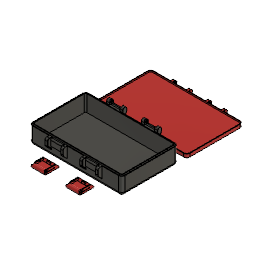
Milwaukee Tool Box Double Lock (Autodesk Fusion 360 design; units mm, degrees)
part number: 2025-08-27-12-33-30-467
Autodesk Fusion 360 part; units mm, degrees
note: some values were not read from the file. Chosen so that the rebuilt part matches the saved one: which bodies a step acts on; that a step has no effect; which face or edge a step refers to. Set by a fixed rule: which sketch regions a step uses.
sketch "Box" plane through (0, 0, 0) normal (0, 0, 1) x (1, 0, 0)
  line L0 (65.5, 43) -> (-65.5, 43)
  line L1 (-70.5, 38) -> (-70.5, -38)
  line L2 (-65.5, -43) -> (65.5, -43)
  line L3 (70.5, -38) -> (70.5, 38)
  line L4 (70.5, 43) -> (-70.5, -43) construction
  line L5 (-70.5, 43) -> (70.5, -43) construction
  arc A0 (-65.5, 43) -> (-70.5, 38) centre (-65.5, 38) ccw
  arc A1 (70.5, 38) -> (65.5, 43) centre (65.5, 38) ccw
  arc A2 (65.5, -43) -> (70.5, -38) centre (65.5, -38) ccw
  arc A3 (-70.5, -38) -> (-65.5, -43) centre (-65.5, -38) ccw
  line L6 (65.5, 40) -> (-65.5, 40)
  arc A4 (-65.5, 40) -> (-67.5, 38) centre (-65.5, 38) ccw
  line L7 (-67.5, 38) -> (-67.5, -38)
  arc A5 (-67.5, -38) -> (-65.5, -40) centre (-65.5, -38) ccw
  line L8 (-65.5, -40) -> (65.5, -40)
  arc A6 (65.5, -40) -> (67.5, -38) centre (65.5, -38) ccw
  line L9 (67.5, -38) -> (67.5, 38)
  arc A7 (67.5, 38) -> (65.5, 40) centre (65.5, 38) ccw
  line L10 (-68.5, 38) -> (-68.5, -38)
  arc A8 (-68.5, -38) -> (-65.5, -41) centre (-65.5, -38) ccw
  line L11 (-65.5, -41) -> (65.5, -41)
  arc A9 (65.5, -41) -> (68.5, -38) centre (65.5, -38) ccw
  line L12 (68.5, -38) -> (68.5, 38)
  arc A10 (68.5, 38) -> (65.5, 41) centre (65.5, 38) ccw
  line L13 (65.5, 41) -> (-65.5, 41)
  arc A11 (-65.5, 41) -> (-68.5, 38) centre (-65.5, 38) ccw
  dimension "d5" = 141
  dimension "d6" = 86
  dimension "d7" = 5
  dimension "d10" = -3
  dimension "d95" = 1
  constraint horizontal L0
  constraint perpendicular L0 L1
  constraint parallel L0 L2
  constraint parallel L1 L3
  constraint coincident L4 origin
  constraint coincident L5 origin
  constraint coincident L5.start L0
  constraint coincident L5.start L1
  constraint tangent L0 A0
  constraint tangent L1 A0
  constraint coincident L4.start L0
  constraint coincident L4.start L3
  constraint tangent L0 A1
  constraint tangent L3 A1
  constraint coincident L5.end L3
  constraint coincident L5.end L2
  constraint tangent L3 A2
  constraint tangent L2 A2
  constraint equal A1 A2
  constraint coincident L4.end L2
  constraint coincident L4.end L1
  constraint tangent L2 A3
  constraint tangent L1 A3
  constraint equal A0 A1
  constraint equal A0 A3
  measures "d5" distance of L4.end L5.end
  measures "d6" distance of L5.start L4.end
  measures "d7" radius of A0
extrude "Extrude1" add sketch "Box" along normal blind 26 contours L0 L1 L2 L3 A0 A1 A2 A3 makes body 1
extrude "Extrude15" add sketch "Box" along normal blind 27 contours L10 A8 L11 A9 L12 A10 L13 A11 bodies 1
extrude "Extrude2" add sketch "Box" along normal blind 2 contours L6 A4 L7 A5 L8 A6 L9 A7 bodies 1
chamfer "Chamfer7" distance 0.99 angle 45 8 edges at (0, -41, 26) (-67.6213, -40.1213, 26) (-68.5, 0, 26) (-67.6213, 40.1213, 26) (0, 41, 26) (67.6213, 40.1213, 26) (68.5, 0, 26) (67.6213, -40.1213, 26) on bodies 1
chamfer "Chamfer1" distance 3 angle 45 8 edges at (0, -43, 0) (69.0355, -41.5355, 0) (70.5, 0, 0) (69.0355, 41.5355, 0) (0, 43, 0) (-69.0355, 41.5355, 0) (-70.5, 0, 0) (-69.0355, -41.5355, 0) on bodies 1
fillet "Fillet1" radius 4 8 edges at (-69.0355, 41.5355, 3) (0, 43, 3) (69.0355, 41.5355, 3) (70.5, 0, 3) (69.0355, -41.5355, 3) (0, -43, 3) (-69.0355, -41.5355, 3) (-70.5, 0, 3) on bodies 1
sketch "Lid" plane through (0, 0, 26) normal (0, 0, 1) x (-1, 0, 0)
  arc A0 (70.5, 38) -> (65.5, 43) centre (65.5, 38) ccw
  line L0 (65.5, 43) -> (-65.5, 43)
  arc A1 (-65.5, 43) -> (-70.5, 38) centre (-65.5, 38) ccw
  line L1 (-70.5, 38) -> (-70.5, -38)
  arc A2 (-70.5, -38) -> (-65.5, -43) centre (-65.5, -38) ccw
  line L2 (-65.5, -43) -> (65.5, -43)
  arc A3 (65.5, -43) -> (70.5, -38) centre (65.5, -38) ccw
  line L3 (70.5, -38) -> (70.5, 38)
  arc A4 (65.5, -43) -> (70.5, -38) centre (65.5, -38) ccw
  line L4 (-65.5, -43) -> (65.5, -43)
  line L5 (70.5, -38) -> (70.5, 38)
  arc A5 (70.5, 38) -> (65.5, 43) centre (65.5, 38) ccw
  line L6 (65.5, 43) -> (-65.5, 43)
  arc A6 (-65.5, 43) -> (-70.5, 38) centre (-65.5, 38) ccw
  line L7 (-70.5, 38) -> (-70.5, -38)
  arc A7 (-70.5, -38) -> (-65.5, -43) centre (-65.5, -38) ccw
  line L8 (69.6, -38) -> (69.6, 38)
  arc A8 (69.6, 38) -> (65.5, 42.1) centre (65.5, 38) ccw
  line L9 (65.5, 42.1) -> (-65.5, 42.1)
  arc A9 (-65.5, 42.1) -> (-69.6, 38) centre (-65.5, 38) ccw
  line L10 (-69.6, 38) -> (-69.6, -38)
  arc A10 (-69.6, -38) -> (-65.5, -42.1) centre (-65.5, -38) ccw
  line L11 (-65.5, -42.1) -> (65.5, -42.1)
  arc A11 (65.5, -42.1) -> (69.6, -38) centre (65.5, -38) ccw
  arc A12 (-69.49, -38) -> (-65.5, -41.99) centre (-65.5, -38) ccw
  dimension "d18" = -0.9
extrude "Extrude3" add sketch "Lid" along normal blind 6 separate body contours A0 L0 A1 L1 A2 L2 A3 L3 A4 L4 L5 A5 L6 A6 L7 A7 | L8 A8 L9 A9 L10 A10 L11 A11 makes body 2
extrude "Extrude16" cut sketch "Lid" along normal blind 1 contours L8 A8 L9 A9 L10 A10 L11 A11 bodies 2
chamfer "Chamfer8" distance 1 angle 45 16 edges at (-68.3991, 40.8991, 27) (-69.6, 0, 27) (-68.3991, -40.8991, 27) (0, -42.1, 27) (68.3991, -40.8991, 27) (69.6, 0, 27) (68.3991, 40.8991, 27) (0, 42.1, 27) (0, -43, 32) (69.0355, -41.5355, 32) (70.5, 0, 32) (69.0355, 41.5355, 32) (0, 43, 32) (-69.0355, 41.5355, 32) (-70.5, 0, 32) (-69.0355, -41.5355, 32) on bodies 2
sketch "Lid Hinge and Latch" plane through (0, 0, 0) normal (1, 0, 0) x (0, 1, 0)
  circle A0 centre (46.2, 29) radius 1.8
  line L0 (43, 26) -> (46.2, 26)
  circle A1 centre (-46.2, 29) radius 1.8 construction
  line L1 (-44.8771, 27.5) -> (-43.9639, 27)
  circle A2 centre (-46.2, 29) radius 2
  circle A3 centre (-46.2, 29) radius 3
  line L2 (-44.8771, 30.5) -> (-43.9639, 31)
  line L3 (-49.2, 29) -> (-49.2, 9)
  line L4 (-49.2, 9) -> (-47.7, 9)
  line L5 (-47.7, 9) -> (-43, 13.7)
  line L6 (-43, 13.7) -> (-43, 26.4722)
  line L7 (-46.5, 26.015) -> (-46.5, 15.7)
  line L8 (-46.5, 15.7) -> (-43.5, 15.7)
  line L9 (-46, 15.7) -> (-46, 26.0067)
  line L10 (-43.9639, 27) -> (-43, 26.4722)
  line L11 (-43.5, 15.7) -> (-43, 15.2)
  line L12 (-46.5, 15.7) -> (-43.75, 12.95)
  line L13 (43, 26) -> (43, 31)
  line L14 (-43, 4.6569) -> (-43, 26)
  line L15 (43, 4.6569) -> (43, 26)
  line L16 (-49.2, 29) -> (-49.2, 30.2426)
  line L17 (-49.2, 30.2426) -> (-48.3213, 31.1213)
  line L18 (-38, 0) -> (-40, 0)
  line L19 (42, 32) -> (47, 32)
  line L20 (47, 32) -> (47.6938, 31.6017)
  line L21 (43, 31) -> (42, 32)
  circle A4 centre (46.2, 29) radius 3
  line L22 (-43, 26) -> (-43, 31)
  point P0 (-43, 26.4722)
  point P1 (-38, 0)
  point P2 (42, 32)
  dimension "d37" = 3.6
  dimension "d110" = 3.6
  dimension "d111" = 6
  dimension "d112" = 4
  dimension "d113" = 4
  dimension "d114" = 3
  dimension "d120" = 45
  dimension "d121" = 1.5
  dimension "d124" = 3
  dimension "d130" = 0.5
  dimension "d131" = 2
  dimension "d132" = 45
  dimension "d133" = 0.5
  dimension "d277" = 1.2426
  dimension "d337" = 89.2
  dimension "d342" = 29
  dimension "d343" = 9
  dimension "d353" = 5
  dimension "d354" = 29.863
  dimension "d355" = 6
  dimension "d356" = 89.2
  constraint coincident L1.end A3
  constraint coincident L2.end A3
  constraint concentric A1 A2
  constraint coincident L1.start A2
  constraint coincident A1.centre A2.centre
  constraint coincident L2.start A2
  constraint vertical L1.start L2.start
  constraint vertical L2.end L1.end
  constraint vertical L3
  constraint tangent A3 L3
  constraint perpendicular L3 L4
  constraint perpendicular L4 L6
  constraint vertical L7
  constraint vertical L9
  constraint parallel L1 L10
  constraint coincident A3 L7.start
  constraint coincident A3 L9.end
  constraint horizontal L8
  constraint coincident L9.start L8
  constraint coincident L6 L11.end
  constraint coincident L5 L12.end
  constraint perpendicular L5 L12
  constraint coincident A3 L3.start
  constraint coincident P0 L6.end
  constraint coincident P0 L14
  constraint coincident L0.start L13.start
  constraint perpendicular L0 L13
  constraint parallel L3 L16
  constraint coincident A3 L17.end
  constraint coincident L3.start L16.start
  constraint tangent A3 L17
  constraint horizontal L19
  constraint coincident P2 L19.start
  constraint concentric A0 A4
  constraint coincident L0.end A4
  constraint tangent L0 A4
  constraint coincident L20.end A4
  constraint tangent L20 A4
  measures "d37" diameter of A0
  measures "d110" diameter of A1
  measures "d111" diameter of A3
  measures "d112" distance of L2.end L1.end
  measures "d113" diameter of A2
  measures "d114" distance of L1.start L2.start
  measures "d120" angle of L4 L5
  measures "d121" distance of L3.end L4.end
  measures "d124" distance of L6 L9
  measures "d130" distance of L7.end L9.start
  measures "d131" distance of L5.end L8
  measures "d132" angle of L6 L11
  measures "d133" distance of L6 L8.end
  measures "d277" distance of L3.start L16.end
  measures "d337" distance of A1.centre L15
  measures "d342" distance of A1.centre L18
  measures "d343" distance of L4 L18
  measures "d353" distance of P2 L19.end
  measures "d354" angle of L19 L20
  measures "d355" diameter of A4
  measures "d356" distance of A0.centre L22
extrude "Extrude7" add sketch "Lid Hinge and Latch" along normal mid plane 15 from surface at 26.5 separate body contours L0 L13 L19 L21 A4 | A4 | L19 L20 A4 makes body 3
extrude "Extrude8" add sketch "Lid Hinge and Latch" along normal mid plane 18 from surface at 26.5 contours A0 bodies 3
chamfer "Chamfer2" distance 0.5 angle 45 2 faces at (17.5, 46.1024, 28.7514) (35.5, 46.1024, 28.7514) on bodies 3
sketch "Lid Hinge Cut" plane through (0, 43, 0) normal (0, 1, 0) x (-1, 0, 0)
  line L0 (-65.5, 26) -> (65.5, 26)
  line L1 (65.5, 26) -> (65.5, 31)
  line L2 (-65.5, 31) -> (-65.5, 26)
  line L3 (-34, 30.8) -> (-35.5, 29.934) construction
  line L4 (-35.5, 29.934) -> (-35.5, 30.8) construction
  line L5 (-35.5, 30.8) -> (-34, 30.8) construction
  line L6 (-19, 30.8) -> (-17.5, 29.934) construction
  line L7 (-17.5, 29.934) -> (-17.5, 30.8) construction
  line L8 (-17.5, 30.8) -> (-19, 30.8) construction
  line L9 (-35, 30.8) -> (-35, 27.2)
  line L10 (-18, 27.2) -> (-18, 30.8)
  line L11 (-35.5, 27.7) -> (-35.5, 30.3)
  line L12 (-17.5, 30.3) -> (-17.5, 27.7)
  line L13 (65.5, 31) -> (-65.5, 31)
  line L14 (-19, 26) -> (-19, 31)
  line L15 (-34, 31) -> (-34, 26)
  line L16 (-29, 32) -> (-24, 32)
  line L17 (-24, 32) -> (-24, 26)
  line L18 (-24, 26) -> (-29, 26)
  line L19 (-29, 26) -> (-29, 32)
  line L20 (-19, 32) -> (-34, 32)
  dimension "d357" = 30
  dimension "d358" = 30
  dimension "d365" = 5
  dimension "d366" = 5
  constraint perpendicular L0 L4
  constraint perpendicular L4 L5
  constraint perpendicular L0 L7
  constraint perpendicular L7 L8
  constraint coincident L3.end L11
  constraint coincident L6.end L12
  constraint coincident L3.start L15
  constraint coincident L6.start L14
  constraint coincident L5 L9.start
  constraint coincident L8 L10.end
  constraint horizontal L16
  constraint vertical L17
  constraint horizontal L18
  constraint vertical L19
  constraint coincident L0 L17.end
  constraint coincident L16.start L20
  measures "d357" angle of L3 L5
  measures "d358" angle of L6 L8
  measures "d365" distance of L17 L20.start
  measures "d366" distance of L16.start L20.end
extrude "Extrude40" cut sketch "Lid Hinge Cut" along normal through all contours L0 L13 L17 L18 L19 | L13 L16 L17 L19 L20 bodies 3
extrude "Extrude26" add sketch "Lid Hinge and Latch" along normal mid plane 20 from surface at 26.5 separate body contours L1 A2 A3 L2 | A3 L6 L8 L9 L10 L11 L14 L22 | A3 L3 L4 L5 L7 L12 | L5 L6 L8 L11 L12 L14 | A3 L16 L17 picked at (-44.3747, 30.9359) makes body 4
extrude "Extrude27" add sketch "Lid Hinge and Latch" along normal mid plane 17 from surface at 26.5 contours A2 bodies 4
extrude "Extrude28" add sketch "Lid Hinge and Latch" along normal mid plane 18 from surface at 26.5 contours L1 A2 A3 L2 | L1 A2 A3 L2 bodies 4
chamfer "Chamfer14" distance 0.49 angle 45 2 edges at (35, -48.0647, 29.7232) (18, -48.0647, 29.7232) on bodies 4
chamfer "Chamfer15" distance 0.5 angle 45 2 edges at (35.5, -43.2, 29) (17.5, -43.2, 29) on bodies 4
extrude "Extrude29" cut sketch "Lid Hinge and Latch" along normal mid plane 17 from surface at 26.5 contours A3 L6 L8 L9 L10 L11 L14 L22 | L5 L6 L8 L11 L12 L14 bodies 4
extrude "Extrude30" add sketch "Lid Hinge and Latch" along normal mid plane 5 from surface at 26.5 contours L5 L6 L8 L11 L12 L14 bodies 4
chamfer "Chamfer18" distance 0.4 angle 45 3 edges at (35, -43, 20.0861) (18, -43, 20.0861) (26.5, -49.2, 9) on bodies 4
fillet "Fillet4" radius 1 1 edges at (26.5, -47.7, 9) on bodies 4
sketch "Box and Lacth Hinge" plane through (0, 0, 0) normal (1, 0, 0) x (0, 1, 0)
  line L0 (43, 26) -> (43, 18)
  line L1 (-46.2, 32) -> (-42, 32)
  line L2 (-46, 24) -> (-46, 16.2)
  line L3 (-45.5, 15.7) -> (-43, 15.7)
  line L4 (-43, 9) -> (-43, 26)
  line L5 (-46, 16.2) -> (-45.5, 15.7)
  arc A0 (-46.2, 26) -> (-49.2, 23) centre (-46.2, 23) ccw
  line L6 (-49.2, 23) -> (-49.2, 16.8569)
  line L7 (-48.0284, 14.0284) -> (-43, 9)
  line L8 (-45.5, 15.7) -> (-43, 13.2)
  line L9 (43.2, 26) -> (43.2, 29)
  line L10 (48.0284, 23.0284) -> (43, 18)
  arc A1 (-49.2, 16.8569) -> (-48.0284, 14.0284) centre (-45.2, 16.8569) ccw
  circle A2 centre (-46.2, 29) radius 3
  line L11 (-43, 26) -> (-46.2, 26)
  arc A3 (-44, 26) -> (-46, 24) centre (-44, 24) ccw
  line L12 (43, 26) -> (45.0864, 26)
  line L13 (-43, 26) -> (-43, 31)
  circle A4 centre (-46.2, 29) radius 1.8
  arc A5 (48.0284, 23.0284) -> (49.2, 25.8569) centre (45.2, 25.8569) ccw
  line L14 (49.2, 29) -> (49.2, 25.8569)
  circle A6 centre (46.2, 29) radius 2
  circle A7 centre (46.2, 29) radius 1.8 construction
  circle A8 centre (46.2, 29) radius 3
  line L15 (47.7, 30.3229) -> (48.2, 31.2361)
  line L16 (44.7, 30.3229) -> (44.2, 31.2361)
  circle A9 centre (46.2, 29) radius 3.2 construction
  line L17 (43, 26) -> (46.2, 26)
  line L18 (-38, 0) -> (38, 0)
  line L19 (-43, 31) -> (-42, 32)
  line L20 (-46.2, 32) -> (-47, 32)
  line L21 (-47, 32) -> (-47.6938, 31.6017)
  circle A10 centre (46.2, 29) radius 1.3
  line L22 (47.3136, 26) -> (49.2, 26)
  arc A11 (45.0864, 26) -> (47.3136, 26) centre (46.2, 29) ccw
  point P0 (-46, 15.7)
  point P1 (-46, 15.7)
  point P2 (-49.2, 29)
  point P3 (-48.8, 9)
  point P4 (43, 26)
  point P5 (43, 26)
  point P6 (43, 31)
  dimension "d136" = 0.5
  dimension "d137" = 0.5
  dimension "d140" = 3
  dimension "d150" = 45
  dimension "d182" = 45
  dimension "d239" = 4
  dimension "d244" = 3
  dimension "d252" = 2
  dimension "d270" = 4
  dimension "d309" = 3.6
  dimension "d310" = 6
  dimension "d311" = 4
  dimension "d312" = 4
  dimension "d313" = 3
  dimension "d321" = 6.4
  dimension "d352" = 18
  dimension "d363" = 0.8
  constraint vertical L2
  constraint horizontal L3
  constraint vertical L4
  constraint coincident P1 L2
  constraint coincident P1 L3
  constraint horizontal A0.end A0.centre
  constraint vertical L6
  constraint parallel L5 L8
  constraint coincident L4 L3.end
  constraint vertical L9
  constraint coincident L0.end L10.end
  constraint vertical L0
  constraint tangent L6 A1
  constraint tangent L7 A1
  constraint coincident A2 A0.start
  constraint tangent A2 L11
  constraint horizontal L11
  constraint coincident L11 A3.start
  constraint tangent L2 A3
  constraint tangent L11 A3
  constraint coincident P1 P0
  constraint coincident L4 L8.end
  constraint vertical A0.end P2
  constraint coincident L1.start A2
  constraint horizontal L1
  constraint horizontal L4.start P3
  constraint horizontal L12
  constraint coincident P5 P4
  constraint coincident L12 A11.start
  constraint tangent L10 A5
  constraint vertical L14
  constraint coincident A5.end L14.end
  constraint tangent A5 L14
  constraint coincident L15.end A8
  constraint coincident L16.end A8
  constraint concentric A6 A7
  constraint coincident L15.start A6
  constraint coincident L16.start A6
  constraint coincident L9.end A8
  constraint horizontal L9.end A6.centre
  constraint coincident L14.start A8
  constraint concentric A8 A9
  constraint horizontal L14.start A6.centre
  constraint horizontal L15.start L16.start
  constraint horizontal L16.end L15.end
  constraint vertical L1.start A2.centre
  constraint coincident A6.centre A7.centre
  constraint coincident L12 L9.start
  constraint tangent A2 L20
  constraint coincident A2 L21.end
  constraint tangent A2 L21
  constraint coincident L1.end L19.end
  constraint coincident L12.end A9
  constraint coincident A9 L22.start
  constraint coincident L14 L22.end
  constraint perpendicular L14 L22
  constraint horizontal L12.end L22.start
  constraint concentric A9 A11
  measures "d136" distance of P1 L2.end
  measures "d137" distance of P1 L3.start
  measures "d140" distance of L2 L4
  measures "d150" angle of L4 L7
  measures "d182" angle of L0 L10
  measures "d239" radius of A1
  measures "d244" radius of A0
  measures "d252" radius of A3
  measures "d270" radius of A5
  measures "d309" diameter of A7
  measures "d310" diameter of A8
  measures "d311" distance of L16.end L15.end
  measures "d312" diameter of A6
  measures "d313" distance of L15.start L16.start
  measures "d321" diameter of A9
  measures "d352" distance of L0.end L18
  measures "d363" distance of L1.start L20.end
extrude "Extrude11" add sketch "Box and Lacth Hinge" along normal mid plane 25 from surface at 26.5 separate body contours L0 L10 L12 A5 L14 L17 L22 A11 | L9 L12 A8 L17 | A6 A8 L15 L16 | L14 A8 L17 L22 A11 | A6 A8 L15 L16 | A6 | A10 makes body 5
extrude "Extrude10" cut sketch "Box and Lacth Hinge" along normal mid plane 15.4 from surface at 26.5 contours L9 L12 A8 L17 | A6 A8 L15 L16 | L14 A8 L17 L22 A11 | A6 A8 L15 L16 | L1 A2 L11 L13 L19 bodies 5
extrude "Extrude12" cut sketch "Box and Lacth Hinge" along normal mid plane 18.4 from surface at 26.5 contours A6 | A10 bodies 5
extrude "Extrude39" cut sketch "Box and Lacth Hinge" along normal mid plane 17.4 from surface at 26.5 contours A6 A8 L15 L16 picked at (44.5493, 31.0867) bodies 5
chamfer "Chamfer4" distance 0.499 angle 45 2 faces at (17.3, 47.1704, 28.4739) (35.7, 45.9397, 29.8141) on bodies 5
chamfer "Chamfer21" distance 0.5 distance2 0.5 2 edges at (17.8, 46.2, 32) (35.2, 46.2, 32) measured on face at (15.6, 43.8719, 30.892) measured on face at (37.4, 48.5281, 30.892) on bodies 5
chamfer "Chamfer3" distance 0.2 angle 45 10 edges at (14, 46.2, 32) (14, 49.2, 27.4284) (14, 48.8955, 24.3261) (14, 45.5142, 20.5142) (14, 43.2, 27.5) (39, 49.2, 27.4284) (39, 46.2, 32) (39, 43.2, 27.5) (39, 45.5142, 20.5142) (39, 48.8955, 24.3261) on bodies 5
extrude "Extrude31" add sketch "Box and Lacth Hinge" along normal mid plane 28 from surface at 26.5 separate body contours L1 A2 L11 L13 L19 | A2 | A2 L20 L21 | A4 makes body 6
extrude "Extrude32" cut sketch "Box and Lacth Hinge" along normal mid plane 20.4 from surface at 26.5 contours L1 A2 L11 L13 L19 | A2 | A2 L20 L21 bodies 6
extrude "Extrude33" cut sketch "Box and Lacth Hinge" along normal mid plane 17.4 from surface at 26.5 contours A4 bodies 6 makes body 7 at (40.5, -45.1333, 29.6667)
chamfer "Chamfer17" distance 0.5 angle 45 2 edges at (35.2, -47.8782, 28.3491) (17.8, -47.8782, 29.6509) on bodies 6 7
chamfer "Chamfer16" distance 0.2 angle 45 6 edges at (40.5, -49.0987, 28.227) (40.5, -47.3469, 31.8008) (40.5, -44.6, 26) (12.5, -49.0987, 28.227) (12.5, -44.6, 26) (12.5, -47.3469, 31.8008) on bodies 6 7
extrude "Extrude21" add sketch "Box and Lacth Hinge" along normal mid plane 28 from surface at 26.5 separate body contours L2 L4 L5 A0 L6 L7 L8 A1 L11 A3 | L2 L3 L4 L5 L11 A3 | L3 L4 L8 makes body 8
extrude "Extrude22" cut sketch "Box and Lacth Hinge" along normal mid plane 20.4 from surface at 26.5 contours L2 L4 L5 A0 L6 L7 L8 A1 L11 A3 | L2 L3 L4 L5 L11 A3 | L3 L4 L8 bodies 8 makes body 9 at (40.5, -44.6761, 16.3428)
chamfer "Chamfer11" distance 0.2 angle 45 10 edges at (12.5, -49.2, 19.9284) (12.5, -48.3213, 25.1213) (12.5, -44.6, 26) (12.5, -45.5142, 11.5142) (12.5, -48.8955, 15.3261) (40.5, -49.2, 19.9284) (40.5, -48.8955, 15.3261) (40.5, -45.5142, 11.5142) (40.5, -44.6, 26) (40.5, -48.3213, 25.1213) on bodies 8 9
sketch "Latch Side" plane through (0, 0, 0) normal (1, 0, 0) x (0, 1, 0)
  line L0 (-48.0284, 14.0284) -> (-43, 9)
  line L1 (-43, 9) -> (-43, 26)
  arc A0 (-46.2, 26) -> (-49.2, 23) centre (-46.2, 23) ccw
  line L2 (-49.2, 23) -> (-49.2, 16.8569)
  arc A1 (-49.2, 16.8569) -> (-48.0284, 14.0284) centre (-45.2, 16.8569) ccw
  line L3 (-43, 26) -> (-46.2, 26)
  line L4 (-43, 25) -> (-46.2, 25)
  arc A2 (-46.2, 25) -> (-48.2, 23) centre (-46.2, 23) ccw
  line L5 (-48.2, 23) -> (-48.2, 16.8569)
  arc A3 (-48.2, 16.8569) -> (-47.3213, 14.7355) centre (-45.2, 16.8569) ccw
  line L6 (-47.3213, 14.7355) -> (-43, 10.4142)
  dimension "d224" = -1
  constraint coincident L1 L6.end
  constraint coincident L1 L4.start
extrude "Extrude25" cut sketch "Latch Side" along normal mid plane 21.4 from surface at 26.5 contours L1 L4 A2 L5 A3 L6 bodies 8 9
chamfer "Chamfer13" distance 0.49 angle 45 10 edges at (15.8, -44.6, 25) (15.8, -45.1607, 12.5749) (15.8, -47.9716, 15.7088) (15.8, -48.2, 19.9284) (15.8, -47.6142, 24.4142) (37.2, -47.6142, 24.4142) (37.2, -48.2, 19.9284) (37.2, -47.9716, 15.7088) (37.2, -45.1607, 12.5749) (37.2, -44.6, 25) on bodies 8 9
extrude "Extrude19" add sketch "Box and Lacth Hinge" along normal mid plane 16.6 from surface at 26.5 separate body contours L2 L3 L4 L5 L11 A3 | L3 L4 L8 makes body 10
extrude "Extrude20" cut sketch "Box and Lacth Hinge" along normal mid plane 5.6 from surface at 26.5 contours L3 L4 L8 bodies 10
ref_plane "WorkPlane1" through (26.5, -44.5, 19.6) normal (0, 1, 0) x (0, 0, 1)
sketch "Nub" plane through (0, -44.5, 0) normal (0, 1, 0) x (1, 0, 0)
  line L0 (18.2, -20.1) -> (34.8, -20.1)
  line L1 (18.2, -16.2) -> (18.2, -24)
  line L2 (34.8, -24) -> (34.8, -16.2)
  line L3 (18.2, -20.1) -> (17.6, -20.1)
  line L4 (18.6, -21.1) -> (34.4, -21.1)
  line L5 (34.8, -20.1) -> (35.4, -20.1)
  line L6 (17.6, -20.1) -> (35.4, -20.1)
  arc A0 (17.6, -20.1) -> (18.6, -21.1) centre (18.6, -20.1) ccw
  arc A1 (34.4, -21.1) -> (35.4, -20.1) centre (34.4, -20.1) ccw
  arc A2 (17.485, -20.1) -> (18.6, -21.215) centre (18.6, -20.1) ccw
  line L7 (18.6, -21.215) -> (34.4, -21.215)
  arc A3 (34.4, -21.215) -> (35.515, -20.1) centre (34.4, -20.1) ccw
  line L8 (17.485, -20.1) -> (17.6, -20.1)
  line L9 (35.4, -20.1) -> (35.515, -20.1)
  point P0 (26.5, -20.1)
  dimension "d176" = 1
  dimension "d225" = 16.6
  dimension "d226" = 17.8
  dimension "d228" = 1
  dimension "d229" = 1
  dimension "d231" = 0.115
  constraint horizontal L0
  constraint coincident L0.end L2
  constraint midpoint L0.start L1
  constraint perpendicular L1 L3
  constraint perpendicular L2 L4
  constraint horizontal L5
  constraint equal L3 L5
  constraint midpoint L0 P0
  constraint midpoint P0 L6
  constraint tangent L4 A0
  constraint coincident L3.end L6.start
  constraint tangent L4 A1
  constraint parallel L3 L8
  constraint parallel L5 L9
  measures "d176" distance of L0 L4
  measures "d225" distance of L0.start L0.end
  measures "d226" distance of L3.end L5.end
  measures "d228" radius of A0
  measures "d229" radius of A1
revolve "Revolve1" add sketch "Nub" angle 360 about axis through (18.2, -44.5, 20.1) along (1, 0, 0) contours L0 L1 L2 L4 L6 A0 A1 | L1 L3 L6 A0 | L2 L5 L6 A1 bodies 10
revolve "Revolve2" cut sketch "Nub" angle 360 about axis through (18.2, -44.5, 20.1) along (1, 0, 0) contours L1 L3 L6 A0 | L2 L5 L6 A1 | L1 A0 A2 L8 | L2 A1 A3 L9 bodies 4
mirror "Mirror8" about plane through (0, 0, 0) normal (1, 0, 0) of bodies 8 9 4 3 5 10 7 6 makes body 11 at (-22.4, 43, 23.3333) makes body 12 at (-32.3333, 44, 32) makes body 13 at (-12.5, -44.629, 16.4176) makes body 14 at (-40.5, -44.629, 16.4176) makes body 15 at (-27.4333, -43, 22.5667) makes body 16 at (-23.5, -49.2, 15.9333) makes body 17 at (-12.5, -45.1333, 29.7333) makes body 18 at (-40.5, -45.1333, 29.7333)
combine "Combine8" operation add target body 2 tool bodies 17 18 12 3 6 7
combine "Combine9" operation add target body 1 tool bodies 14 13 8 9 5 11 15 10
sketch "Column Divider" plane through (0, 0, 2) normal (0, 0, 1) x (-1, 0, 0)
  arc A0 (-67.5, -38) -> (-65.5, -40) centre (-65.5, -38) ccw
  line L0 (-65.5, -40) -> (65.5, -40)
  arc A1 (65.5, -40) -> (67.5, -38) centre (65.5, -38) ccw
  line L1 (67.5, -38) -> (67.5, 38)
  arc A2 (67.5, 38) -> (65.5, 40) centre (65.5, 38) ccw
  line L2 (65.5, 40) -> (-65.5, 40)
  arc A3 (-65.5, 40) -> (-67.5, 38) centre (-65.5, 38) ccw
  line L3 (-67.5, 38) -> (-67.5, -38)
  line L4 (68.5, -41) -> (68.5, 41)
  line L5 (67.5, 1) -> (69.5, 1)
  line L6 (69.5, 1) -> (69.5, -1)
  line L7 (69.5, -1) -> (67.5, -1)
  line L8 (67.5, -1) -> (67.5, 1)
  line L9 (67.5, 1) -> (69.5, -1) construction
  line L10 (69.5, 1) -> (67.5, -1) construction
  point P0 (65.5, 41)
  point P1 (68.5, 38)
  point P2 (65.5, -41)
  point P3 (68.5, -38)
  point P4 (68.5, 0)
  dimension "d344" = 2
  dimension "d345" = 2
  constraint vertical L4
  constraint horizontal L4.start P2
  constraint horizontal L4.end P0
  constraint coincident L4 P1
  constraint horizontal L5
  constraint perpendicular L5 L6
  constraint parallel L5 L7
  constraint parallel L6 L8
  constraint coincident L9 P4
  constraint coincident L10 P4
  constraint midpoint L4 P4
  measures "d344" distance of L6.end L7.end
  measures "d345" distance of L5.end L6.end
extrude "Extrude35" add sketch "Column Divider" along normal blind 25 thin wall 2 centred separate body open curves L4 makes body 19
extrude "Extrude41" add sketch "Column Divider" against normal blind 2 contours L1 L4 L5 L7 L8 | L4 L5 L6 L7 bodies 19
pattern_linear "R-Pattern1" [no effect]
delete_body "RemoveBody1" bodies 19
sketch "Row Divider" plane through (0, 0, 2) normal (0, 0, 1) x (-1, 0, 0)
  arc A0 (-67.5, -38) -> (-65.5, -40) centre (-65.5, -38) ccw
  line L0 (-65.5, -40) -> (65.5, -40)
  arc A1 (65.5, -40) -> (67.5, -38) centre (65.5, -38) ccw
  line L1 (67.5, -38) -> (67.5, 38)
  arc A2 (67.5, 38) -> (65.5, 40) centre (65.5, 38) ccw
  line L2 (65.5, 40) -> (-65.5, 40)
  arc A3 (-65.5, 40) -> (-67.5, 38) centre (-65.5, 38) ccw
  line L3 (-67.5, 38) -> (-67.5, -38)
  line L4 (68.5, 41) -> (-68.5, 41)
  line L5 (-1, 42) -> (1, 42)
  line L6 (1, 42) -> (1, 40)
  line L7 (1, 40) -> (-1, 40)
  line L8 (-1, 40) -> (-1, 42)
  line L9 (-1, 42) -> (1, 40) construction
  line L10 (1, 42) -> (-1, 40) construction
  point P0 (65.5, 41)
  point P1 (68.5, 38)
  point P2 (-68.5, 38)
  point P3 (0, 41)
  dimension "d348" = 2
  dimension "d349" = 2
  constraint horizontal L4
  constraint coincident L4 P0
  constraint vertical L4.start P1
  constraint vertical L4.end P2
  constraint horizontal L5
  constraint perpendicular L5 L6
  constraint parallel L5 L7
  constraint parallel L6 L8
  constraint coincident L9 P3
  constraint coincident L10 P3
  constraint midpoint L4 P3
  measures "d348" distance of L6.end L7.end
  measures "d349" distance of L5.end L6.end
extrude "Extrude36" add sketch "Row Divider" along normal blind 25 thin wall 2 centred separate body open curves L4 makes body 20
extrude "Extrude42" add sketch "Row Divider" against normal blind 2 contours L2 L4 L6 L7 L8 | L4 L5 L6 L8 bodies 20
pattern_linear "R-Pattern2" [no effect]
delete_body "RemoveBody2" bodies 20
sketch "DeWALT Logo" plane through (0, 0, 32) normal (0, 0, 1) x (-1, 0, 0)
  line L0 (-40.5, 42) -> (-65.5, 42)
  arc A0 (-65.5, 42) -> (-69.5, 38) centre (-65.5, 38) ccw
  line L1 (-69.5, 38) -> (-69.5, -38)
  arc A1 (-69.5, -38) -> (-65.5, -42) centre (-65.5, -38) ccw
  line L2 (-34, -42) -> (-34, -47)
  line L3 (-34, -47) -> (-29, -47)
  line L4 (-29, -47) -> (-29, -43)
  line L5 (-29, -43) -> (-24, -43)
  line L6 (-24, -43) -> (-24, -47)
  line L7 (-24, -47) -> (-19, -47)
  line L8 (-19, -47) -> (-19, -42)
  line L9 (19, -42) -> (19, -47)
  line L10 (19, -47) -> (24, -47)
  line L11 (24, -47) -> (24, -43)
  line L12 (24, -43) -> (29, -43)
  line L13 (29, -43) -> (29, -47)
  line L14 (29, -47) -> (34, -47)
  line L15 (34, -47) -> (34, -42)
  arc A2 (65.5, -42) -> (69.5, -38) centre (65.5, -38) ccw
  line L16 (69.5, -38) -> (69.5, 38)
  arc A3 (69.5, 38) -> (65.5, 42) centre (65.5, 38) ccw
  line L17 (-36.2996, 43) -> (39.3068, 43) construction
  line L18 (39.3068, 43) -> (39.3068, -43) construction
  line L19 (39.3068, -43) -> (-39.3068, -43) construction
  line L20 (-39.3068, -43) -> (-36.2996, 43) construction
  line L21 (-36.2996, 43) -> (39.3068, -43) construction
  line L22 (39.3068, 43) -> (-39.3068, -43) construction
  line L23 (-38.5614, -7.1361) -> (-18.7971, 0.3781)
  line L24 (-18.7971, 0.3781) -> (-19.9348, -2.109)
  line L25 (-19.9348, -2.109) -> (6.8411, 7.0456)
  line L26 (6.8411, 7.0456) -> (5.3594, 3.9764)
  line L27 (5.3594, 3.9764) -> (36.4479, 15.9091)
  line L28 (36.4479, 15.9091) -> (13.0852, 10.0618)
  line L29 (13.0852, 10.0618) -> (15.0167, 13.7395)
  line L30 (15.0167, 13.7395) -> (-13.9287, 2.971)
  line L31 (-13.9287, 2.971) -> (-12.2883, 6.1725)
  line L32 (-12.2883, 6.1725) -> (-38.5614, -7.1361)
  line L33 (19.0119, -13.0363) -> (22.425, -10.1523)
  spline S0 degree 2 poles (22.425, -10.1523) (23.7744, -11.6869) (23.9067, -11.7928) knots 0 0 0 1 1 1
  spline S1 degree 2 poles (23.9067, -11.7928) (24.0125, -11.6869) (26.8171, -9.3057) knots 0 0 0 1 1 1
  line L34 (26.8171, -9.3057) -> (26.4202, -13.248)
  line L35 (26.4202, -13.248) -> (36.4479, -4.8342)
  line L36 (36.4479, -4.8342) -> (29.5952, -8.115)
  line L37 (29.5952, -8.115) -> (31.3415, 6.6487)
  spline S2 degree 2 poles (31.3415, 6.6487) (29.2513, 8.2097) (29.0661, 8.3156) knots 0 0 0 1 1 1
  spline S3 degree 3 poles (29.0661, 8.3156) (28.8808, 6.9133) (27.1875, -6.6069) (27.1081, -7.3478) knots 0 0 0 0 1 1 1 1
  line L38 (27.1081, -7.3478) -> (27.1081, -7.3742)
  line L39 (27.1081, -7.3742) -> (25.1238, -9.0411)
  line L40 (25.1238, -9.0411) -> (24.7004, -8.6178)
  line L41 (24.7004, -8.6178) -> (26.2879, 4.8495)
  spline S4 degree 2 poles (26.2879, 4.8495) (24.1448, 6.437) (24.0125, 6.5429) knots 0 0 0 1 1 1
  spline S5 degree 3 poles (24.0125, 6.5429) (23.9861, 6.4106) (22.5573, -5.7867) (22.2398, -8.6971) knots 0 0 0 0 1 1 1 1
  line L42 (22.2398, -8.6971) -> (20.2819, -10.364)
  line L43 (20.2819, -10.364) -> (19.8585, -9.9407)
  line L44 (19.8585, -9.9407) -> (21.3931, 3.1827)
  line L45 (21.3931, 3.1827) -> (19.1177, 4.8495)
  line L46 (19.1177, 4.8495) -> (17.2656, -11.1313)
  line L47 (17.2656, -11.1313) -> (19.0119, -13.0363)
  line L48 (13.4292, -10.0994) -> (15.8104, -9.7025)
  line L49 (15.8104, -9.7025) -> (16.1015, -7.3742)
  line L50 (16.1015, -7.3742) -> (13.7467, -7.824)
  line L51 (13.7467, -7.824) -> (13.4292, -10.0994)
  line L52 (0.7292, -9.1205) -> (1.6817, -1.765)
  line L53 (1.6817, -1.765) -> (2.2108, -1.2094)
  line L54 (2.2108, -1.2094) -> (3.084, -1.9503)
  line L55 (3.084, -1.9503) -> (2.2108, -8.8559)
  line L56 (2.2108, -8.8559) -> (4.5656, -8.2738)
  line L57 (4.5656, -8.2738) -> (5.4917, -1.0771)
  line L58 (5.4917, -1.0771) -> (6.1796, -0.1511)
  line L59 (6.1796, -0.1511) -> (6.9204, -0.8125)
  line L60 (6.9204, -0.8125) -> (6.0473, -8.0621)
  line L61 (6.0473, -8.0621) -> (8.4286, -7.5594)
  line L62 (8.4286, -7.5594) -> (9.2223, -0.9713)
  line L63 (9.2223, -0.9713) -> (10.2013, 0.3781)
  line L64 (10.2013, 0.3781) -> (10.8892, -0.204)
  line L65 (10.8892, -0.204) -> (9.3546, -12.5865)
  line L66 (9.3546, -12.5865) -> (11.6829, -12.2161)
  line L67 (11.6829, -12.2161) -> (13.1117, -0.3098)
  line L68 (13.1117, -0.3098) -> (14.2758, 1.3041)
  line L69 (14.2758, 1.3041) -> (14.8844, 0.8279)
  line L70 (14.8844, 0.8279) -> (13.879, -6.4217)
  line L71 (13.879, -6.4217) -> (16.2602, -5.9455)
  line L72 (16.2602, -5.9455) -> (17.345, 2.4683)
  line L73 (17.345, 2.4683) -> (15.2813, 4.1087)
  line L74 (15.2813, 4.1087) -> (13.2175, 1.3306)
  line L75 (13.2175, 1.3306) -> (11.0744, 3.0504)
  line L76 (11.0744, 3.0504) -> (9.0106, 0.2458)
  line L77 (9.0106, 0.2458) -> (6.7881, 2.1508)
  line L78 (6.7881, 2.1508) -> (4.6186, -0.7332)
  line L79 (4.6186, -0.7332) -> (2.8458, 0.8279)
  line L80 (2.8458, 0.8279) -> (-0.2233, -2.5059)
  line L81 (-0.2233, -2.5059) -> (-1.1758, -9.5438)
  line L82 (-1.1758, -9.5438) -> (0.7292, -9.1205)
  line L83 (-31.7881, -9.438) -> (-31.1002, -10.02)
  line L84 (-31.1002, -10.02) -> (-31.2325, -11.1313)
  line L85 (-31.2325, -11.1313) -> (-34.4075, -12.9305)
  line L86 (-34.4075, -12.9305) -> (-31.841, -16.1055)
  line L87 (-31.841, -16.1055) -> (-29.4862, -14.0682)
  line L88 (-29.4862, -14.0682) -> (-28.9306, -9.6496)
  line L89 (-28.9306, -9.6496) -> (-25.8085, -7.9298)
  line L90 (-25.8085, -7.9298) -> (-25.0677, -8.5384)
  line L91 (-25.0677, -8.5384) -> (-25.2264, -9.729)
  line L92 (-25.2264, -9.729) -> (-28.6925, -11.634)
  line L93 (-28.6925, -11.634) -> (-25.9408, -15.0207)
  line L94 (-25.9408, -15.0207) -> (-23.4008, -12.8511)
  line L95 (-23.4008, -12.8511) -> (-22.8717, -8.6442)
  line L96 (-22.8717, -8.6442) -> (-21.7339, -7.5594)
  line L97 (-21.7339, -7.5594) -> (-19.9612, -11.0784)
  line L98 (-19.9612, -11.0784) -> (-23.93, -14.7032)
  line L99 (-23.93, -14.7032) -> (-22.1308, -14.4386)
  line L100 (-22.1308, -14.4386) -> (-19.1146, -11.8986)
  line L101 (-19.1146, -11.8986) -> (-19.8289, -17.6136)
  line L102 (-19.8289, -17.6136) -> (-17.6594, -17.3225)
  line L103 (-17.6594, -17.3225) -> (-16.4687, -7.5065)
  line L104 (-16.4687, -7.5065) -> (-15.1458, -6.0513)
  line L105 (-15.1458, -6.0513) -> (-14.8283, -6.3159)
  line L106 (-14.8283, -6.3159) -> (-15.6221, -12.5336)
  line L107 (-15.6221, -12.5336) -> (-13.2937, -12.0044)
  line L108 (-13.2937, -12.0044) -> (-12.5529, -6.3688)
  line L109 (-12.5529, -6.3688) -> (-11.521, -5.1253)
  line L110 (-11.521, -5.1253) -> (-11.0712, -5.5221)
  line L111 (-11.0712, -5.5221) -> (-11.865, -11.6869)
  line L112 (-11.865, -11.6869) -> (-9.5102, -11.2107)
  line L113 (-9.5102, -11.2107) -> (-8.7694, -5.4428)
  line L114 (-8.7694, -5.4428) -> (-7.6846, -4.0669)
  line L115 (-7.6846, -4.0669) -> (-7.2083, -4.4903)
  line L116 (-7.2083, -4.4903) -> (-8.0285, -10.9461)
  line L117 (-8.0285, -10.9461) -> (-5.6737, -10.4434)
  line L118 (-5.6737, -10.4434) -> (-5.6208, -9.9407)
  line L119 (-5.6208, -9.9407) -> (-3.9804, -10.7344)
  line L120 (-3.9804, -10.7344) -> (-1.6785, -7.7975)
  line L121 (-1.6785, -7.7975) -> (-1.0171, -2.5323)
  line L122 (-1.0171, -2.5323) -> (-3.2396, -0.6273)
  line L123 (-3.2396, -0.6273) -> (-5.2769, -3.2732)
  line L124 (-5.2769, -3.2732) -> (-7.0231, -1.7915)
  line L125 (-7.0231, -1.7915) -> (-8.9546, -4.2521)
  line L126 (-8.9546, -4.2521) -> (-10.595, -2.7969)
  line L127 (-10.595, -2.7969) -> (-12.3942, -5.1782)
  line L128 (-12.3942, -5.1782) -> (-14.114, -3.67)
  line L129 (-14.114, -3.67) -> (-16.4423, -6.21)
  line L130 (-16.4423, -6.21) -> (-18.215, -4.8078)
  line L131 (-18.215, -4.8078) -> (-18.7442, -9.1205)
  line L132 (-18.7442, -9.1205) -> (-20.6227, -5.284)
  line L133 (-20.6227, -5.284) -> (-23.1098, -7.6917)
  line L134 (-23.1098, -7.6917) -> (-24.7237, -6.3423)
  line L135 (-24.7237, -6.3423) -> (-29.5127, -8.9882)
  line L136 (-29.5127, -8.9882) -> (-30.7298, -7.9298)
  line L137 (-30.7298, -7.9298) -> (-35.1483, -10.4963)
  line L138 (-35.1483, -10.4963) -> (-35.2806, -11.4488)
  line L139 (-35.2806, -11.4488) -> (-31.7881, -9.438)
  line L140 (-31.6558, -14.2798) -> (-32.6877, -13.0628)
  line L141 (-32.6877, -13.0628) -> (-31.4177, -12.3484)
  line L142 (-31.4177, -12.3484) -> (-31.6558, -14.2798)
  line L143 (-25.7027, -13.0628) -> (-26.8139, -11.7663)
  line L144 (-26.8139, -11.7663) -> (-25.4117, -10.999)
  line L145 (-25.4117, -10.999) -> (-25.7027, -13.0628)
  line L146 (-4.88, -4.2786) -> (-3.9275, -3.1144)
  line L147 (-3.9275, -3.1144) -> (-3.4248, -3.5642)
  line L148 (-3.4248, -3.5642) -> (-4.1921, -9.6761)
  line L149 (-4.1921, -9.6761) -> (-5.4885, -8.9882)
  line L150 (-5.4885, -8.9882) -> (-4.88, -4.2786)
  line L151 (-65.5, -42) -> (-34, -42)
  line L152 (40.3, 47) -> (36.7, 47)
  line L153 (12.7, 47) -> (12.5, 46.5983)
  line L154 (12.5, 46.5983) -> (12.5, 42)
  line L155 (12.5, 42) -> (-12.5, 42)
  line L156 (-12.5, 42) -> (-12.5, 46.5983)
  line L157 (-12.5, 46.5983) -> (-12.7, 47)
  line L158 (-19, -42) -> (19, -42)
  line L159 (34, -42) -> (65.5, -42)
  line L160 (65.5, 42) -> (40.5, 42)
  line L161 (40.5, 42) -> (40.5, 46.5983)
  line L162 (40.5, 46.5983) -> (40.3, 47)
  line L163 (36.7, 47) -> (36.7, 42)
  line L164 (36.7, 42) -> (16.3, 42)
  line L165 (16.3, 42) -> (16.3, 47)
  line L166 (16.3, 47) -> (12.7, 47)
  line L167 (-12.7, 47) -> (-16.3, 47)
  line L168 (-16.3, 47) -> (-16.3, 42)
  line L169 (-16.3, 42) -> (-36.7, 42)
  line L170 (-36.7, 42) -> (-36.7, 47)
  line L171 (-36.7, 47) -> (-40.3, 47)
  line L172 (-40.3, 47) -> (-40.5, 46.5983)
  line L173 (-40.5, 46.5983) -> (-40.5, 42)
  point P0 (-65.5, -43)
  point P1 (-65.5, 43)
  constraint horizontal L17
  constraint perpendicular L17 L18
  constraint parallel L17 L19
  constraint horizontal L19.end P0
  constraint coincident origin L22
  constraint horizontal L17.start P1
extrude "Extrude43" add sketch "DeWALT Logo" against normal blind 0.6 separate body contours L23 L24 L25 L26 L27 L28 L29 L30 L31 L32 | L33 S0 S1 L34 L35 L36 L37 S2 S3 L38 L39 L40 L41 S4 S5 L42 L43 L44 L45 L46 L47 | L48 L49 L50 L51 | L52 L53 L54 L55 L56 L57 L58 L59 L60 L61 L62 L63 L64 L65 L66 L67 L68 L69 L70 L71 L72 L73 L74 L75 L76 L77 L78 L79 L80 L81 L82 | L83 L84 L85 L86 L87 L88 L89 L90 L91 L92 L93 L94 L95 L96 L97 L98 L99 L100 L101 L102 L103 L104 L105 L106 L107 L108 L109 L110 L111 L112 L113 L114 L115 L116 L117 L118 L119 L120 L121 L122 L123 L124 L125 L126 L127 L128 L129 L130 L131 L132 L133 L134 L135 L136 L137 L138 L139 makes body 21 at (-15.2195, 8.3003, 32) makes body 22 at (-16.1632, 0.8831, 32) makes body 23 at (6.9085, 8.1415, 32) makes body 24 at (-29.3483, 2.938, 32) makes body 25 at (-2.643, -7.9187, 32)
scale "Scale1" factor 1 about (0, 0, 32) bodies 21 22 23 25 24
combine "Combine10" operation cut target body 2 tool bodies 21 22 23 25 24 keep tools
move_body "Move4" bodies 4 16 to x (1, 0, 0) y (0, 0, 1) z (0, -1, 0) at (0, -17.2, 75.2)
move_body "Move5" bodies 4 16 to x (1, 0, 0) y (0, 1, 0) z (0, 0, 1) at (0, -25, -26)
move_body "Move8" bodies 2 21 22 23 24 25 to x (1, 0, 0) y (0, -1, 0) z (0, 0, -1) at (0, 84, 64)
move_body "Move7" bodies 2 21 22 23 24 25 to x (1, 0, 0) y (0, 1, 0) z (0, 0, 1) at (0, 15, -32)
equation "Width = ( ( SlotWidth + 2 mm ) * Rows ) + 4 mm"
equation "Length = ( ( SlotLength + 2 mm ) * Columns ) + 4 mm"
equation "Height = SlotHeight + 8 mm"
equation "ConrnerRadius = 5 mm"
equation "d5 = Length"
equation "d6 = Width"
equation "d7 = ConrnerRadius"
equation "d11 = Height - 7 mm"
equation "HingePosition = ( HingesDistance / 2 ) + 14 mm"
equation "d46 = HingePosition"
equation "d47 = HingeSize"
equation "d49 = HingePosition"
equation "d50 = HingeSize + 3 mm"
equation "d61 = HingePosition"
equation "d62 = HingeSize + 0.4 mm"
equation "d64 = HingePosition"
equation "d65 = HingeSize + 10 mm"
equation "d67 = HingePosition"
equation "d68 = HingeSize + 3.4 mm"
equation "HingesDistance = ( Length - ( ConrnerRadius * 2 ) - 56 mm ) / 3"
equation "d97 = Height - 6 mm"
equation "d147 = HingePosition"
equation "d148 = LatchSize - 3.4 mm"
equation "d152 = HingePosition"
equation "d155 = HingePosition"
equation "d156 = LatchSize + 8 mm"
equation "d158 = HingePosition"
equation "d159 = LatchSize + 0.4 mm"
equation "d171 = HingePosition"
equation "d172 = LatchSize + 1.4 mm"
equation "HingeSize = 15 mm"
equation "LatchSize = 20 mm"
equation "d187 = HingePosition"
equation "d188 = LatchSize"
equation "d190 = HingePosition"
equation "d191 = LatchSize - 3 mm"
equation "d193 = HingePosition"
equation "d194 = LatchSize - 2 mm"
equation "d198 = HingePosition"
equation "d199 = LatchSize - 3 mm"
equation "d201 = HingePosition"
equation "d209 = HingePosition"
equation "d210 = LatchSize + 8 mm"
equation "d212 = HingePosition"
equation "d213 = LatchSize + 0.4 mm"
equation "d215 = HingePosition"
equation "d216 = LatchSize - 2.6 mm"
equation "d226 = LatchSize - 2.2 mm"
equation "d257 = -Height + 7 mm"
equation "d261 = -Height + 1 mm"
equation "d279 = Height - 8 mm"
equation "RowSectionDistance = ( Width - 4 mm ) / Rows"
equation "ColumnSectionDistance = ( Length - 4 mm ) / Columns"
equation "d283 = Columns"
equation "d285 = ColumnSectionDistance"
equation "d288 = Height - 8 mm"
equation "d290 = Rows"
equation "d292 = RowSectionDistance"
equation "Rows = 1"
equation "Columns = 1"
equation "d324 = HingePosition"
equation "d325 = HingeSize + 2.4 mm"
equation "d337 = Width + 3.2 mm"
equation "SlotWidth = 80 mm"
equation "SlotLength = 135 mm"
equation "SlotHeight = 25 mm"
equation "d342 = Height - 4 mm"
equation "d343 = Height - 24 mm"
equation "d352 = Height - 15 mm"
equation "d356 = Width + 3.2 mm"
equation "LogoWidth = 75 mm"
equation "d438 = LogoWidth / 75 mm"
equation "d437 = LogoWidth"
named bodies: "Box", "Lid", "Body8 (1)", "Body9 (1)", "Body12 (1)", "Body14 (1)", "Body16 (1)", "Body18 (1)", "Body20 (1)", "Body25 (1)", "Body27 (1)", "Body29 (1)", "Body30 (1)", "Body30 (2)", "Body31 (1)", "Body31 (1) (1)", "Latch 1", "Lid Hinge", "Latch 2"
